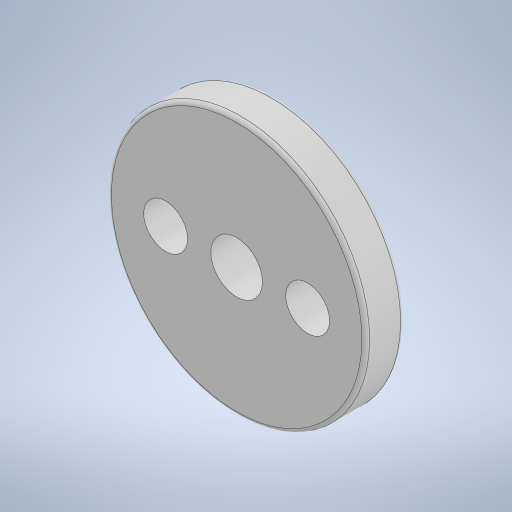
# Autodesk Inventor part: homemade_setcolor
Saved by Autodesk Inventor 2024 (Build 280153000, 153)
## iProperties
Created: 2025-04-19
Part Number: homemade_setcolor
Material: 一般
Document SubType Name: Modeling
Designer: 1412z
Density: 1 g/cm^3
Appearance: 既定
Author: 1412z
Autodesk Inventor part; units mm, degrees
ref_plane "YZ Plane" through (0, 0, 0) normal (1, 0, 0) x (0, 1, 0)
ref_plane "XZ Plane" through (0, 0, 0) normal (0, 1, 0) x (-1, 0, 0)
ref_plane "XY Plane" through (0, 0, 0) normal (0, 0, 1) x (1, 0, 0)
sketch "スケッチ1" plane through (0, 0, 0) normal (0, 0, 1) x (1, 0, 0)
  circle A0 centre (0, 0) radius 10
  circle A1 centre (0, 0) radius 2
  dimension "d0" = 20
  dimension "d1" = 4
  constraints: 2 centre point, 2 coincident
  measures "d0" diameter of A0
  measures "d1" diameter of A1
extrude "押し出し1" add sketch "スケッチ1" along normal blind 3
sketch "スケッチ2" plane through (0, 0, 3) normal (0, 0, 1) x (1, 0, 0)
  circle A0 centre (0, 0) radius 5.5
  circle A1 centre (-5.5, 0) radius 1.7
  circle A2 centre (5.5, 0) radius 1.7
  dimension "d4" = 11
  dimension "d5" = 3.4
  dimension "d6" = 3.4
  constraints: 3 centre point, 2 point on circle, 1 coincident
  measures "d4" diameter of A0
  measures "d5" diameter of A1
  measures "d6" diameter of A2
extrude "押し出し2" cut sketch "スケッチ2" against normal blind 3 contours A0 A2 | A0 A2 | A1 A0 | A0 A1
fillet "フィレット1" radius 0.3 2 edges at (-10, 0, 3) (-10, 0, 0)
